Autodesk Fusion 360 part; units mm, degrees
(part 3 of 3)
sketch "Sketch1 (2)" plane through (0, 0, 12.7) normal (0, 0, 1) x (-1, 0, 0)
  arc A0 (-5.2324, 8.6498) -> (-8.6498, 5.2324) centre (0, 0) ccw
  arc A1 (-10.637, 4.5964) -> (-8.6498, 5.2324) centre (-10.0081, 6.054) ccw
  line L0 (-10.637, 4.5964) -> (-21.9128, 9.4616)
  spline S0 degree 5 poles (-21.9128, 9.4616) (-21.9552, 9.4799) (-22.0407, 9.5141) (-22.1712, 9.5583) (-22.3491, 9.6037) (-22.5768, 9.6426) (-22.8081, 9.6692) (-23.0414, 9.6889) (-23.2758, 9.7048) (-23.5109, 9.7174) (-23.7467, 9.7262) (-23.9837, 9.7295) (-24.2219, 9.7262) (-24.4615, 9.7158) (-24.7023, 9.6987) (-24.9439, 9.6758) (-25.1862, 9.648) (-25.4288, 9.6159) (-25.6717, 9.5798) (-25.9149, 9.5397) (-26.1582, 9.4952) (-26.4018, 9.4462) (-26.6456, 9.3926) (-26.8896, 9.3344) (-27.1337, 9.2719) (-27.3777, 9.2051) (-27.6217, 9.1343) (-27.8655, 9.0596) (-28.109, 8.9811) (-28.3523, 8.8987) (-28.5954, 8.8125) (-28.838, 8.7225) (-29.0803, 8.6286) (-29.3222, 8.531) (-29.5637, 8.4296) (-29.8046, 8.3246) (-30.045, 8.216) (-30.2848, 8.1038) (-30.5239, 7.9882) (-30.7623, 7.869) (-31.0001, 7.7465) (-31.2371, 7.6205) (-31.4733, 7.491) (-31.7087, 7.3583) (-31.9432, 7.2221) (-32.1769, 7.0827) (-32.4096, 6.9401) (-32.6414, 6.7942) (-32.8722, 6.6451) (-33.1019, 6.4928) (-33.3306, 6.3374) (-33.5583, 6.1789) (-33.7848, 6.0173) (-34.0102, 5.8526) (-34.2343, 5.6849) (-34.4573, 5.5142) (-34.6791, 5.3405) (-34.8996, 5.1639) (-35.1188, 4.9843) (-35.3367, 4.8018) (-35.5532, 4.6165) (-35.7684, 4.4283) (-35.9823, 4.2373) (-36.1947, 4.0436) (-36.4056, 3.847) (-36.6151, 3.6477) (-36.823, 3.4457) (-37.0294, 3.241) (-37.2343, 3.0337) (-37.4376, 2.8237) (-37.6393, 2.6111) (-37.7995, 2.4389) (-37.9189, 2.3086) (-37.9982, 2.2212) (-38.0377, 2.1774) knots 0 0 0 0 0 0 0.01428571 0.02857143 0.04285714 0.05714286 0.07142857 0.08571429 0.1 0.11428571 0.12857143 0.14285714 0.15714286 0.17142857 0.18571429 0.2 0.21428571 0.22857143 0.24285714 0.25714286 0.27142857 0.28571429 0.3 0.31428571 0.32857143 0.34285714 0.35714286 0.37142857 0.38571429 0.4 0.41428571 0.42857143 0.44285714 0.45714286 0.47142857 0.48571429 0.5 0.51428571 0.52857143 0.54285714 0.55714286 0.57142857 0.58571429 0.6 0.61428571 0.62857143 0.64285714 0.65714286 0.67142857 0.68571429 0.7 0.71428571 0.72857143 0.74285714 0.75714286 0.77142857 0.78571429 0.8 0.81428571 0.82857143 0.84285714 0.85714286 0.87142857 0.88571429 0.9 0.91428571 0.92857143 0.94285714 0.95714286 0.97142857 0.98571429 1 1 1 1 1 1
  arc A2 (-38.0377, 2.1774) -> (-38.0377, -2.1774) centre (0, 0) ccw
  spline S1 degree 5 poles (-38.0377, -2.1774) (-37.9982, -2.2212) (-37.9189, -2.3086) (-37.7995, -2.4389) (-37.6393, -2.6111) (-37.4376, -2.8237) (-37.2343, -3.0337) (-37.0294, -3.241) (-36.823, -3.4457) (-36.6151, -3.6477) (-36.4056, -3.847) (-36.1947, -4.0436) (-35.9823, -4.2373) (-35.7684, -4.4283) (-35.5532, -4.6165) (-35.3367, -4.8018) (-35.1188, -4.9843) (-34.8996, -5.1639) (-34.6791, -5.3405) (-34.4573, -5.5142) (-34.2343, -5.6849) (-34.0102, -5.8526) (-33.7848, -6.0173) (-33.5583, -6.1789) (-33.3306, -6.3374) (-33.1019, -6.4928) (-32.8722, -6.6451) (-32.6414, -6.7942) (-32.4096, -6.9401) (-32.1769, -7.0827) (-31.9432, -7.2221) (-31.7087, -7.3583) (-31.4733, -7.491) (-31.2371, -7.6205) (-31.0001, -7.7465) (-30.7623, -7.869) (-30.5239, -7.9882) (-30.2848, -8.1038) (-30.045, -8.216) (-29.8046, -8.3246) (-29.5637, -8.4296) (-29.3222, -8.531) (-29.0803, -8.6286) (-28.838, -8.7225) (-28.5954, -8.8125) (-28.3523, -8.8987) (-28.109, -8.9811) (-27.8655, -9.0596) (-27.6217, -9.1343) (-27.3777, -9.2051) (-27.1337, -9.2719) (-26.8896, -9.3344) (-26.6456, -9.3926) (-26.4018, -9.4462) (-26.1582, -9.4952) (-25.9149, -9.5397) (-25.6717, -9.5798) (-25.4288, -9.6159) (-25.1862, -9.648) (-24.9439, -9.6758) (-24.7023, -9.6987) (-24.4615, -9.7158) (-24.2219, -9.7262) (-23.9837, -9.7295) (-23.7467, -9.7262) (-23.5109, -9.7174) (-23.2758, -9.7048) (-23.0414, -9.6889) (-22.8081, -9.6692) (-22.5768, -9.6426) (-22.3491, -9.6037) (-22.1712, -9.5583) (-22.0407, -9.5141) (-21.9552, -9.4799) (-21.9128, -9.4616) knots -1 -1 -1 -1 -1 -1 -0.98571429 -0.97142857 -0.95714286 -0.94285714 -0.92857143 -0.91428571 -0.9 -0.88571429 -0.87142857 -0.85714286 -0.84285714 -0.82857143 -0.81428571 -0.8 -0.78571429 -0.77142857 -0.75714286 -0.74285714 -0.72857143 -0.71428571 -0.7 -0.68571429 -0.67142857 -0.65714286 -0.64285714 -0.62857143 -0.61428571 -0.6 -0.58571429 -0.57142857 -0.55714286 -0.54285714 -0.52857143 -0.51428571 -0.5 -0.48571429 -0.47142857 -0.45714286 -0.44285714 -0.42857143 -0.41428571 -0.4 -0.38571429 -0.37142857 -0.35714286 -0.34285714 -0.32857143 -0.31428571 -0.3 -0.28571429 -0.27142857 -0.25714286 -0.24285714 -0.22857143 -0.21428571 -0.2 -0.18571429 -0.17142857 -0.15714286 -0.14285714 -0.12857143 -0.11428571 -0.1 -0.08571429 -0.07142857 -0.05714286 -0.04285714 -0.02857143 -0.01428571 0 0 0 0 0 0
  line L1 (-21.9128, -9.4616) -> (-10.637, -4.5964)
  arc A3 (-8.6498, -5.2324) -> (-10.637, -4.5964) centre (-10.0081, -6.054) ccw
  arc A4 (-8.6498, -5.2324) -> (-5.2324, -8.6498) centre (0, 0) ccw
  arc A5 (-4.5964, -10.637) -> (-5.2324, -8.6498) centre (-6.054, -10.0081) ccw
  line L2 (-4.5964, -10.637) -> (-9.4616, -21.9128)
  spline S2 degree 5 poles (-9.4616, -21.9128) (-9.4799, -21.9552) (-9.5141, -22.0407) (-9.5583, -22.1712) (-9.6037, -22.3491) (-9.6426, -22.5768) (-9.6692, -22.8081) (-9.6889, -23.0414) (-9.7048, -23.2758) (-9.7174, -23.5109) (-9.7262, -23.7467) (-9.7295, -23.9837) (-9.7262, -24.2219) (-9.7158, -24.4615) (-9.6987, -24.7023) (-9.6758, -24.9439) (-9.648, -25.1862) (-9.6159, -25.4288) (-9.5798, -25.6717) (-9.5397, -25.9149) (-9.4952, -26.1582) (-9.4462, -26.4018) (-9.3926, -26.6456) (-9.3344, -26.8896) (-9.2719, -27.1337) (-9.2051, -27.3777) (-9.1343, -27.6217) (-9.0596, -27.8655) (-8.9811, -28.109) (-8.8987, -28.3523) (-8.8125, -28.5954) (-8.7225, -28.838) (-8.6286, -29.0803) (-8.531, -29.3222) (-8.4296, -29.5637) (-8.3246, -29.8046) (-8.216, -30.045) (-8.1038, -30.2848) (-7.9882, -30.5239) (-7.869, -30.7623) (-7.7465, -31.0001) (-7.6205, -31.2371) (-7.491, -31.4733) (-7.3583, -31.7087) (-7.2221, -31.9432) (-7.0827, -32.1769) (-6.9401, -32.4096) (-6.7942, -32.6414) (-6.6451, -32.8722) (-6.4928, -33.1019) (-6.3374, -33.3306) (-6.1789, -33.5583) (-6.0173, -33.7848) (-5.8526, -34.0102) (-5.6849, -34.2343) (-5.5142, -34.4573) (-5.3405, -34.6791) (-5.1639, -34.8996) (-4.9843, -35.1188) (-4.8018, -35.3367) (-4.6165, -35.5532) (-4.4283, -35.7684) (-4.2373, -35.9823) (-4.0436, -36.1947) (-3.847, -36.4056) (-3.6477, -36.6151) (-3.4457, -36.823) (-3.241, -37.0294) (-3.0337, -37.2343) (-2.8237, -37.4376) (-2.6111, -37.6393) (-2.4389, -37.7995) (-2.3086, -37.9189) (-2.2212, -37.9982) (-2.1774, -38.0377) knots 0 0 0 0 0 0 0.01428571 0.02857143 0.04285714 0.05714286 0.07142857 0.08571429 0.1 0.11428571 0.12857143 0.14285714 0.15714286 0.17142857 0.18571429 0.2 0.21428571 0.22857143 0.24285714 0.25714286 0.27142857 0.28571429 0.3 0.31428571 0.32857143 0.34285714 0.35714286 0.37142857 0.38571429 0.4 0.41428571 0.42857143 0.44285714 0.45714286 0.47142857 0.48571429 0.5 0.51428571 0.52857143 0.54285714 0.55714286 0.57142857 0.58571429 0.6 0.61428571 0.62857143 0.64285714 0.65714286 0.67142857 0.68571429 0.7 0.71428571 0.72857143 0.74285714 0.75714286 0.77142857 0.78571429 0.8 0.81428571 0.82857143 0.84285714 0.85714286 0.87142857 0.88571429 0.9 0.91428571 0.92857143 0.94285714 0.95714286 0.97142857 0.98571429 1 1 1 1 1 1
  arc A6 (-2.1774, -38.0377) -> (2.1774, -38.0377) centre (0, 0) ccw
  spline S3 degree 5 poles (2.1774, -38.0377) (2.2212, -37.9982) (2.3086, -37.9189) (2.4389, -37.7995) (2.6111, -37.6393) (2.8237, -37.4376) (3.0337, -37.2343) (3.241, -37.0294) (3.4457, -36.823) (3.6477, -36.6151) (3.847, -36.4056) (4.0436, -36.1947) (4.2373, -35.9823) (4.4283, -35.7684) (4.6165, -35.5532) (4.8018, -35.3367) (4.9843, -35.1188) (5.1639, -34.8996) (5.3405, -34.6791) (5.5142, -34.4573) (5.6849, -34.2343) (5.8526, -34.0102) (6.0173, -33.7848) (6.1789, -33.5583) (6.3374, -33.3306) (6.4928, -33.1019) (6.6451, -32.8722) (6.7942, -32.6414) (6.9401, -32.4096) (7.0827, -32.1769) (7.2221, -31.9432) (7.3583, -31.7087) (7.491, -31.4733) (7.6205, -31.2371) (7.7465, -31.0001) (7.869, -30.7623) (7.9882, -30.5239) (8.1038, -30.2848) (8.216, -30.045) (8.3246, -29.8046) (8.4296, -29.5637) (8.531, -29.3222) (8.6286, -29.0803) (8.7225, -28.838) (8.8125, -28.5954) (8.8987, -28.3523) (8.9811, -28.109) (9.0596, -27.8655) (9.1343, -27.6217) (9.2051, -27.3777) (9.2719, -27.1337) (9.3344, -26.8896) (9.3926, -26.6456) (9.4462, -26.4018) (9.4952, -26.1582) (9.5397, -25.9149) (9.5798, -25.6717) (9.6159, -25.4288) (9.648, -25.1862) (9.6758, -24.9439) (9.6987, -24.7023) (9.7158, -24.4615) (9.7262, -24.2219) (9.7295, -23.9837) (9.7262, -23.7467) (9.7174, -23.5109) (9.7048, -23.2758) (9.6889, -23.0414) (9.6692, -22.8081) (9.6426, -22.5768) (9.6037, -22.3491) (9.5583, -22.1712) (9.5141, -22.0407) (9.4799, -21.9552) (9.4616, -21.9128) knots -1 -1 -1 -1 -1 -1 -0.98571429 -0.97142857 -0.95714286 -0.94285714 -0.92857143 -0.91428571 -0.9 -0.88571429 -0.87142857 -0.85714286 -0.84285714 -0.82857143 -0.81428571 -0.8 -0.78571429 -0.77142857 -0.75714286 -0.74285714 -0.72857143 -0.71428571 -0.7 -0.68571429 -0.67142857 -0.65714286 -0.64285714 -0.62857143 -0.61428571 -0.6 -0.58571429 -0.57142857 -0.55714286 -0.54285714 -0.52857143 -0.51428571 -0.5 -0.48571429 -0.47142857 -0.45714286 -0.44285714 -0.42857143 -0.41428571 -0.4 -0.38571429 -0.37142857 -0.35714286 -0.34285714 -0.32857143 -0.31428571 -0.3 -0.28571429 -0.27142857 -0.25714286 -0.24285714 -0.22857143 -0.21428571 -0.2 -0.18571429 -0.17142857 -0.15714286 -0.14285714 -0.12857143 -0.11428571 -0.1 -0.08571429 -0.07142857 -0.05714286 -0.04285714 -0.02857143 -0.01428571 0 0 0 0 0 0
  line L3 (9.4616, -21.9128) -> (4.5964, -10.637)
  arc A7 (5.2324, -8.6498) -> (4.5964, -10.637) centre (6.054, -10.0081) ccw
  arc A8 (5.2324, -8.6498) -> (8.6498, -5.2324) centre (0, 0) ccw
  arc A9 (10.637, -4.5964) -> (8.6498, -5.2324) centre (10.0081, -6.054) ccw
  line L4 (10.637, -4.5964) -> (21.9128, -9.4616)
  spline S4 degree 5 poles (21.9128, -9.4616) (21.9552, -9.4799) (22.0407, -9.5141) (22.1712, -9.5583) (22.3491, -9.6037) (22.5768, -9.6426) (22.8081, -9.6692) (23.0414, -9.6889) (23.2758, -9.7048) (23.5109, -9.7174) (23.7467, -9.7262) (23.9837, -9.7295) (24.2219, -9.7262) (24.4615, -9.7158) (24.7023, -9.6987) (24.9439, -9.6758) (25.1862, -9.648) (25.4288, -9.6159) (25.6717, -9.5798) (25.9149, -9.5397) (26.1582, -9.4952) (26.4018, -9.4462) (26.6456, -9.3926) (26.8896, -9.3344) (27.1337, -9.2719) (27.3777, -9.2051) (27.6217, -9.1343) (27.8655, -9.0596) (28.109, -8.9811) (28.3523, -8.8987) (28.5954, -8.8125) (28.838, -8.7225) (29.0803, -8.6286) (29.3222, -8.531) (29.5637, -8.4296) (29.8046, -8.3246) (30.045, -8.216) (30.2848, -8.1038) (30.5239, -7.9882) (30.7623, -7.869) (31.0001, -7.7465) (31.2371, -7.6205) (31.4733, -7.491) (31.7087, -7.3583) (31.9432, -7.2221) (32.1769, -7.0827) (32.4096, -6.9401) (32.6414, -6.7942) (32.8722, -6.6451) (33.1019, -6.4928) (33.3306, -6.3374) (33.5583, -6.1789) (33.7848, -6.0173) (34.0102, -5.8526) (34.2343, -5.6849) (34.4573, -5.5142) (34.6791, -5.3405) (34.8996, -5.1639) (35.1188, -4.9843) (35.3367, -4.8018) (35.5532, -4.6165) (35.7684, -4.4283) (35.9823, -4.2373) (36.1947, -4.0436) (36.4056, -3.847) (36.6151, -3.6477) (36.823, -3.4457) (37.0294, -3.241) (37.2343, -3.0337) (37.4376, -2.8237) (37.6393, -2.6111) (37.7995, -2.4389) (37.9189, -2.3086) (37.9982, -2.2212) (38.0377, -2.1774) knots 0 0 0 0 0 0 0.01428571 0.02857143 0.04285714 0.05714286 0.07142857 0.08571429 0.1 0.11428571 0.12857143 0.14285714 0.15714286 0.17142857 0.18571429 0.2 0.21428571 0.22857143 0.24285714 0.25714286 0.27142857 0.28571429 0.3 0.31428571 0.32857143 0.34285714 0.35714286 0.37142857 0.38571429 0.4 0.41428571 0.42857143 0.44285714 0.45714286 0.47142857 0.48571429 0.5 0.51428571 0.52857143 0.54285714 0.55714286 0.57142857 0.58571429 0.6 0.61428571 0.62857143 0.64285714 0.65714286 0.67142857 0.68571429 0.7 0.71428571 0.72857143 0.74285714 0.75714286 0.77142857 0.78571429 0.8 0.81428571 0.82857143 0.84285714 0.85714286 0.87142857 0.88571429 0.9 0.91428571 0.92857143 0.94285714 0.95714286 0.97142857 0.98571429 1 1 1 1 1 1
  arc A10 (38.0377, -2.1774) -> (38.0377, 2.1774) centre (0, 0) ccw
  spline S5 degree 5 poles (38.0377, 2.1774) (37.9982, 2.2212) (37.9189, 2.3086) (37.7995, 2.4389) (37.6393, 2.6111) (37.4376, 2.8237) (37.2343, 3.0337) (37.0294, 3.241) (36.823, 3.4457) (36.6151, 3.6477) (36.4056, 3.847) (36.1947, 4.0436) (35.9823, 4.2373) (35.7684, 4.4283) (35.5532, 4.6165) (35.3367, 4.8018) (35.1188, 4.9843) (34.8996, 5.1639) (34.6791, 5.3405) (34.4573, 5.5142) (34.2343, 5.6849) (34.0102, 5.8526) (33.7848, 6.0173) (33.5583, 6.1789) (33.3306, 6.3374) (33.1019, 6.4928) (32.8722, 6.6451) (32.6414, 6.7942) (32.4096, 6.9401) (32.1769, 7.0827) (31.9432, 7.2221) (31.7087, 7.3583) (31.4733, 7.491) (31.2371, 7.6205) (31.0001, 7.7465) (30.7623, 7.869) (30.5239, 7.9882) (30.2848, 8.1038) (30.045, 8.216) (29.8046, 8.3246) (29.5637, 8.4296) (29.3222, 8.531) (29.0803, 8.6286) (28.838, 8.7225) (28.5954, 8.8125) (28.3523, 8.8987) (28.109, 8.9811) (27.8655, 9.0596) (27.6217, 9.1343) (27.3777, 9.2051) (27.1337, 9.2719) (26.8896, 9.3344) (26.6456, 9.3926) (26.4018, 9.4462) (26.1582, 9.4952) (25.9149, 9.5397) (25.6717, 9.5798) (25.4288, 9.6159) (25.1862, 9.648) (24.9439, 9.6758) (24.7023, 9.6987) (24.4615, 9.7158) (24.2219, 9.7262) (23.9837, 9.7295) (23.7467, 9.7262) (23.5109, 9.7174) (23.2758, 9.7048) (23.0414, 9.6889) (22.8081, 9.6692) (22.5768, 9.6426) (22.3491, 9.6037) (22.1712, 9.5583) (22.0407, 9.5141) (21.9552, 9.4799) (21.9128, 9.4616) knots -1 -1 -1 -1 -1 -1 -0.98571429 -0.97142857 -0.95714286 -0.94285714 -0.92857143 -0.91428571 -0.9 -0.88571429 -0.87142857 -0.85714286 -0.84285714 -0.82857143 -0.81428571 -0.8 -0.78571429 -0.77142857 -0.75714286 -0.74285714 -0.72857143 -0.71428571 -0.7 -0.68571429 -0.67142857 -0.65714286 -0.64285714 -0.62857143 -0.61428571 -0.6 -0.58571429 -0.57142857 -0.55714286 -0.54285714 -0.52857143 -0.51428571 -0.5 -0.48571429 -0.47142857 -0.45714286 -0.44285714 -0.42857143 -0.41428571 -0.4 -0.38571429 -0.37142857 -0.35714286 -0.34285714 -0.32857143 -0.31428571 -0.3 -0.28571429 -0.27142857 -0.25714286 -0.24285714 -0.22857143 -0.21428571 -0.2 -0.18571429 -0.17142857 -0.15714286 -0.14285714 -0.12857143 -0.11428571 -0.1 -0.08571429 -0.07142857 -0.05714286 -0.04285714 -0.02857143 -0.01428571 0 0 0 0 0 0
  line L5 (21.9128, 9.4616) -> (10.637, 4.5964)
  arc A11 (8.6498, 5.2324) -> (10.637, 4.5964) centre (10.0081, 6.054) ccw
  arc A12 (8.6498, 5.2324) -> (5.2324, 8.6498) centre (0, 0) ccw
  arc A13 (4.5964, 10.637) -> (5.2324, 8.6498) centre (6.054, 10.0081) ccw
  line L6 (4.5964, 10.637) -> (9.4616, 21.9128)
  spline S6 degree 5 poles (9.4616, 21.9128) (9.4799, 21.9552) (9.5141, 22.0407) (9.5583, 22.1712) (9.6037, 22.3491) (9.6426, 22.5768) (9.6692, 22.8081) (9.6889, 23.0414) (9.7048, 23.2758) (9.7174, 23.5109) (9.7262, 23.7467) (9.7295, 23.9837) (9.7262, 24.2219) (9.7158, 24.4615) (9.6987, 24.7023) (9.6758, 24.9439) (9.648, 25.1862) (9.6159, 25.4288) (9.5798, 25.6717) (9.5397, 25.9149) (9.4952, 26.1582) (9.4462, 26.4018) (9.3926, 26.6456) (9.3344, 26.8896) (9.2719, 27.1337) (9.2051, 27.3777) (9.1343, 27.6217) (9.0596, 27.8655) (8.9811, 28.109) (8.8987, 28.3523) (8.8125, 28.5954) (8.7225, 28.838) (8.6286, 29.0803) (8.531, 29.3222) (8.4296, 29.5637) (8.3246, 29.8046) (8.216, 30.045) (8.1038, 30.2848) (7.9882, 30.5239) (7.869, 30.7623) (7.7465, 31.0001) (7.6205, 31.2371) (7.491, 31.4733) (7.3583, 31.7087) (7.2221, 31.9432) (7.0827, 32.1769) (6.9401, 32.4096) (6.7942, 32.6414) (6.6451, 32.8722) (6.4928, 33.1019) (6.3374, 33.3306) (6.1789, 33.5583) (6.0173, 33.7848) (5.8526, 34.0102) (5.6849, 34.2343) (5.5142, 34.4573) (5.3405, 34.6791) (5.1639, 34.8996) (4.9843, 35.1188) (4.8018, 35.3367) (4.6165, 35.5532) (4.4283, 35.7684) (4.2373, 35.9823) (4.0436, 36.1947) (3.847, 36.4056) (3.6477, 36.6151) (3.4457, 36.823) (3.241, 37.0294) (3.0337, 37.2343) (2.8237, 37.4376) (2.6111, 37.6393) (2.4389, 37.7995) (2.3086, 37.9189) (2.2212, 37.9982) (2.1774, 38.0377) knots 0 0 0 0 0 0 0.01428571 0.02857143 0.04285714 0.05714286 0.07142857 0.08571429 0.1 0.11428571 0.12857143 0.14285714 0.15714286 0.17142857 0.18571429 0.2 0.21428571 0.22857143 0.24285714 0.25714286 0.27142857 0.28571429 0.3 0.31428571 0.32857143 0.34285714 0.35714286 0.37142857 0.38571429 0.4 0.41428571 0.42857143 0.44285714 0.45714286 0.47142857 0.48571429 0.5 0.51428571 0.52857143 0.54285714 0.55714286 0.57142857 0.58571429 0.6 0.61428571 0.62857143 0.64285714 0.65714286 0.67142857 0.68571429 0.7 0.71428571 0.72857143 0.74285714 0.75714286 0.77142857 0.78571429 0.8 0.81428571 0.82857143 0.84285714 0.85714286 0.87142857 0.88571429 0.9 0.91428571 0.92857143 0.94285714 0.95714286 0.97142857 0.98571429 1 1 1 1 1 1
  arc A14 (2.1774, 38.0377) -> (-2.1774, 38.0377) centre (0, 0) ccw
  spline S7 degree 5 poles (-2.1774, 38.0377) (-2.2212, 37.9982) (-2.3086, 37.9189) (-2.4389, 37.7995) (-2.6111, 37.6393) (-2.8237, 37.4376) (-3.0337, 37.2343) (-3.241, 37.0294) (-3.4457, 36.823) (-3.6477, 36.6151) (-3.847, 36.4056) (-4.0436, 36.1947) (-4.2373, 35.9823) (-4.4283, 35.7684) (-4.6165, 35.5532) (-4.8018, 35.3367) (-4.9843, 35.1188) (-5.1639, 34.8996) (-5.3405, 34.6791) (-5.5142, 34.4573) (-5.6849, 34.2343) (-5.8526, 34.0102) (-6.0173, 33.7848) (-6.1789, 33.5583) (-6.3374, 33.3306) (-6.4928, 33.1019) (-6.6451, 32.8722) (-6.7942, 32.6414) (-6.9401, 32.4096) (-7.0827, 32.1769) (-7.2221, 31.9432) (-7.3583, 31.7087) (-7.491, 31.4733) (-7.6205, 31.2371) (-7.7465, 31.0001) (-7.869, 30.7623) (-7.9882, 30.5239) (-8.1038, 30.2848) (-8.216, 30.045) (-8.3246, 29.8046) (-8.4296, 29.5637) (-8.531, 29.3222) (-8.6286, 29.0803) (-8.7225, 28.838) (-8.8125, 28.5954) (-8.8987, 28.3523) (-8.9811, 28.109) (-9.0596, 27.8655) (-9.1343, 27.6217) (-9.2051, 27.3777) (-9.2719, 27.1337) (-9.3344, 26.8896) (-9.3926, 26.6456) (-9.4462, 26.4018) (-9.4952, 26.1582) (-9.5397, 25.9149) (-9.5798, 25.6717) (-9.6159, 25.4288) (-9.648, 25.1862) (-9.6758, 24.9439) (-9.6987, 24.7023) (-9.7158, 24.4615) (-9.7262, 24.2219) (-9.7295, 23.9837) (-9.7262, 23.7467) (-9.7174, 23.5109) (-9.7048, 23.2758) (-9.6889, 23.0414) (-9.6692, 22.8081) (-9.6426, 22.5768) (-9.6037, 22.3491) (-9.5583, 22.1712) (-9.5141, 22.0407) (-9.4799, 21.9552) (-9.4616, 21.9128) knots -1 -1 -1 -1 -1 -1 -0.98571429 -0.97142857 -0.95714286 -0.94285714 -0.92857143 -0.91428571 -0.9 -0.88571429 -0.87142857 -0.85714286 -0.84285714 -0.82857143 -0.81428571 -0.8 -0.78571429 -0.77142857 -0.75714286 -0.74285714 -0.72857143 -0.71428571 -0.7 -0.68571429 -0.67142857 -0.65714286 -0.64285714 -0.62857143 -0.61428571 -0.6 -0.58571429 -0.57142857 -0.55714286 -0.54285714 -0.52857143 -0.51428571 -0.5 -0.48571429 -0.47142857 -0.45714286 -0.44285714 -0.42857143 -0.41428571 -0.4 -0.38571429 -0.37142857 -0.35714286 -0.34285714 -0.32857143 -0.31428571 -0.3 -0.28571429 -0.27142857 -0.25714286 -0.24285714 -0.22857143 -0.21428571 -0.2 -0.18571429 -0.17142857 -0.15714286 -0.14285714 -0.12857143 -0.11428571 -0.1 -0.08571429 -0.07142857 -0.05714286 -0.04285714 -0.02857143 -0.01428571 0 0 0 0 0 0
  line L7 (-9.4616, 21.9128) -> (-4.5964, 10.637)
  arc A15 (-5.2324, 8.6498) -> (-4.5964, 10.637) centre (-6.054, 10.0081) ccw
  circle A16 centre (0, 0) radius 6.35
  circle A17 centre (0, 0) radius 7
  circle A18 centre (0, 0) radius 6.35
  line L8 (1.4, -6.8586) -> (1.4, -5.1)
  line L9 (1.4, -5.1) -> (-1.4, -5.1)
  line L10 (-1.4, -5.1) -> (-1.4, -6.8586)
  line L11 (0, -9) -> (0, 8.2774)
  point P0 (0, -7)
  dimension "d17" = 14
  dimension "d18" = 2.8
  dimension "d19" = 1.9
  constraint coincident A0.centre A2.centre
  constraint coincident A17 L8.start
  constraint vertical L8
  constraint perpendicular L8 L9
  constraint coincident A17 L10.end
  constraint perpendicular L9 L10
  constraint perpendicular L9 L11
  constraint symmetric L8 L10 L11
  constraint coincident A17 P0
  constraint coincident L11 P0
  constraint coincident A0.centre L11
  measures "d17" diameter of A17
  measures "d18" distance of L8 L10
  measures "d19" distance of L9 P0
extrude "Extrude3" cut sketch "Sketch1 (2)" against normal blind 12.7 contours A16 A17 A18 L8 L11 | A16 A17 A18 L10 L11 | A16 A17 A18 L8 L11 | A16 A17 A18 L10 L11 in component "Spur Gear (4 teeth)"
extrude "Extrude4" add sketch "Sketch1 (2)" against normal up to surface (12.7 mm away) contours A16 A17 A18 L8 L11 | A16 A18 L8 L9 L11 | A16 A18 L9 L10 L11 | A16 A17 A18 L10 L11 picked at (1.2459, -6.4442) picked at (0.7792, -5.4935) picked at (-0.7792, -5.4935) picked at (-1.2459, -6.4442) in component "Spur Gear (4 teeth)"
component "Spur Gear (4 teeth)" placed x (1, 0, 0) y (0, 1, 0) z (0, 0, 1) at (0, 0, 0)

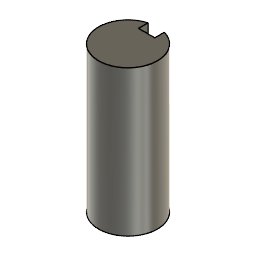
design "Motor Shaft"
Autodesk Fusion 360 part; units mm, degrees
sketch "Sketch1" plane through (0, 0, 0) normal (0, 0, 1) x (1, 0, 0)
  circle A0 centre (0, 0) radius 5.45
  line L0 (0, 7.5) -> (0, -6)
  line L1 (-1.5, 5.2395) -> (-1.5, 3.45)
  line L2 (-1.5, 3.45) -> (1.5, 3.45)
  line L3 (1.5, 3.45) -> (1.5, 5.2395)
  circle A1 centre (0, 0) radius 3.2
  line L4 (-2.0805, -2.4314) -> (2.0805, -2.4314)
  point P0 (0, 5.45)
  dimension "d1" = 10.9
  dimension "d2" = 2
  dimension "d3" = 3
  dimension "d4" = 6.4
  dimension "d5" = 4.161
  constraint coincident A0.centre A1.centre
  constraint vertical L0
  constraint coincident A0 L1.start
  constraint parallel L0 L1
  constraint perpendicular L1 L2
  constraint coincident A0 L3.end
  constraint perpendicular L2 L3
  constraint symmetric L0 L1 L3
  constraint coincident A0 P0
  constraint coincident L0 P0
  constraint coincident A0.centre L0
  constraint coincident A1 L4.start
  constraint coincident A1 L4.end
  constraint perpendicular L0 L4
  measures "d1" diameter of A0
  measures "d2" distance of L2 P0
  measures "d3" distance of L1 L3
  measures "d4" diameter of A1
  measures "d5" distance of L4.start L4.end
extrude "Extrude1" add sketch "Sketch1" along normal blind 15
extrude "Extrude2" add sketch "Sketch1" against normal blind 12 contours A0 L0 L2 L3 A1 | A0 L0 L2 L3 | A0 L0 L1 L2 A1 | A0 L0 L1 L2 | L0 A1 L4 | L0 A1 L4 picked at (-0.1505, -2.9331) picked at (0.1505, -2.9331)
extrude "Extrude3" cut sketch "Sketch1" against normal blind 10 from surface at 15 contours A0 L0 L2 L3 | A0 L0 L1 L2

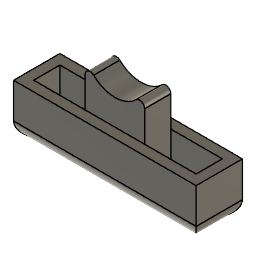
design "Cap 3"
Autodesk Fusion 360 part; units mm, degrees
sketch "Sketch1" plane through (0, 0, 0) normal (0, 0, 1) x (1, 0, 0)
  line L0 (0, 0) -> (32.2, 0)
  line L1 (32.2, 0) -> (32.2, 5.2)
  line L2 (32.2, 5.2) -> (0, 5.2)
  line L3 (0, 5.2) -> (0, 0)
  line L4 (-2, -2) -> (34.2, -2)
  line L5 (34.2, -2) -> (34.2, 7.2)
  line L6 (34.2, 7.2) -> (-2, 7.2)
  line L7 (-2, 7.2) -> (-2, -2)
  line L8 (10.2, 5.2) -> (22, 5.2)
  line L9 (22, 5.2) -> (22, 0)
  line L10 (22, 0) -> (10.2, 0)
  line L11 (10.2, 0) -> (10.2, 5.2)
  dimension "d1" = 5.2
  dimension "d2" = 32.2
  dimension "d3" = 2
  dimension "d4" = 10.2
  dimension "d5" = 10.2
  constraint horizontal L0
  constraint vertical L1
  constraint horizontal L2
  constraint vertical L3
  constraint coincident L0.start L3.end
  constraint horizontal L8
  constraint vertical L9
  constraint horizontal L10
  constraint vertical L11
  constraint coincident L0 L9.end
  constraint coincident L2 L8.start
  measures "d1" distance of L0 L2
  measures "d2" distance of L1 L3
  measures "d4" distance of L3 L11
  measures "d5" distance of L1 L9
extrude "Extrude1" add sketch "Sketch1" along normal blind 8
extrude "Extrude2" add sketch "Sketch1" against normal blind 2 contours L0 L2 L3 L11 | L0 L2 L8 L9 L10 L11 | L0 L1 L2 L9 | L4 L5 L6 L7
extrude "Extrude3" add sketch "Sketch1" along normal blind 18 contours L0 L2 L8 L9 L10 L11
sketch "Sketch2" plane through (0, 5.2, 0) normal (0, 1, 0) x (-1, 0, 0)
  line L0 (-22, 8) -> (-10.2, 8)
  line L1 (-10.2, 8) -> (-10.2, 18)
  line L2 (-10.2, 18) -> (-22, 18)
  line L3 (-22, 18) -> (-22, 8)
  arc A0 (-22, 18) -> (-10.2, 18) centre (-16.1, 19.0909) ccw
  dimension "d19" = 6
  constraint coincident L2.end L3.start
  constraint coincident L1.end L2.start
  measures "d19" radius of A0
extrude "Extrude4" cut sketch "Sketch2" against normal up to surface (5.2 mm away) contours L2 A0
fillet "Fillet1" radius 3 4 edges at (-2, 2.6, -2) (16.1, 7.2, -2) (34.2, 2.6, -2) (16.1, -2, -2)
fillet "Fillet3" radius 1 2 edges at (10.2, 2.6, 18) (22, 2.6, 18)

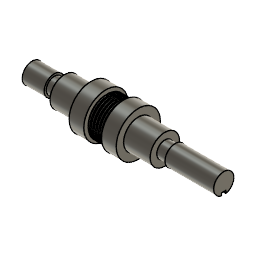
design "Roller 1"
Autodesk Fusion 360 part; units mm, degrees
sketch "Sketch1" plane through (0, 0, 0) normal (1, 0, 0) x (0, 1, 0)
  circle A0 centre (0, 0) radius 10
  circle A1 centre (0, 0) radius 5.5
  circle A2 centre (0, 0) radius 6.9
  line L0 (-1.5, -6.735) -> (-1.5, -4.9)
  line L1 (-1.5, -4.9) -> (1.5, -4.9)
  line L2 (1.5, -4.9) -> (1.5, -6.735)
  line L3 (0, -11) -> (0, 11)
  line L4 (1.0311, 3.6) -> (1.4, 3.6)
  line L5 (1.4, 3.6) -> (1.4, 5.3188)
  line L6 (-1.0311, 3.6) -> (-1.4, 3.6)
  line L7 (-1.4, 3.6) -> (-1.4, 5.3188)
  line L8 (1.0311, 3.6) -> (-1.0311, 3.6)
  circle A3 centre (0, 0) radius 7.9
  circle A4 centre (0, 0) radius 15
  circle A5 centre (0, 0) radius 13
  circle A6 centre (0, 0) radius 12
  point P0 (0, -6.9)
  point P1 (0, 5.5)
  dimension "d1" = 20
  dimension "d4" = -4.5
  dimension "d11" = 13.8
  dimension "d15" = 3
  dimension "d16" = 2
  dimension "d31" = 2.8
  dimension "d32" = 1.9
  dimension "d55" = 1
  dimension "d56" = 5
  dimension "d57" = -2
  dimension "d58" = -1
  constraint coincident A0.centre A1.centre
  constraint coincident A2 L0.start
  constraint vertical L0
  constraint perpendicular L0 L1
  constraint coincident A2 L2.end
  constraint perpendicular L1 L2
  constraint vertical L3
  constraint symmetric L0 L2 L3
  constraint coincident A2 P0
  constraint coincident L3 P0
  constraint coincident A0.centre L3
  constraint horizontal L4
  constraint vertical L5
  constraint coincident A1 L5.end
  constraint horizontal L6
  constraint vertical L7
  constraint coincident A1 L7.end
  constraint perpendicular L3 L8
  constraint coincident L3 P1
  constraint coincident A1 P1
  constraint symmetric L3 L5 L7
  measures "d1" diameter of A0
  measures "d11" diameter of A2
  measures "d15" distance of L0 L2
  measures "d16" distance of L1 P0
  measures "d31" distance of L5 L7
  measures "d32" distance of L8 P1
extrude "Extrude1" add sketch "Sketch1" along normal blind 130 contours A0 L3 A3 | A0 L3 A3 | A2 L3 A3 | A2 L3 A3 | A1 A2 L0 L3 | A1 A2 L2 L3 | A1 A2 L2 L3 | A1 A2 L0 L3 | A1 L3 L6 L7 L8 | A1 L3 L4 L5 L8 | A1 L1 L2 L3 | A1 L0 L1 L3 | A1 L0 L1 L3 L6 L7 L8 | A1 L1 L2 L3 L4 L5 L8
extrude "Extrude2" cut sketch "Sketch1" along normal blind 7 from surface at 15 contours A0 L3 A3 | A0 L3 A3 | A2 L3 A3 | A2 L3 A3 | A1 A2 L0 L3 | A1 A2 L2 L3 | A1 A2 L2 L3 | A1 A2 L0 L3
extrude "Extrude3" cut sketch "Sketch1" along normal blind 7 from surface at 90 contours A0 L3 A3 | A0 L3 A3 | A2 L3 A3 | A2 L3 A3 | A1 A2 L0 L3 | A1 A2 L2 L3 | A1 A2 L2 L3 | A1 A2 L0 L3
extrude "Extrude4" cut sketch "Sketch1" along normal up to surface (33 mm away) from surface at 97 contours A0 L3 A3 | A0 L3 A3 | A2 L3 A3 | A2 L3 A3
extrude "Extrude5" cut sketch "Sketch1" along normal up to surface (24 mm away) from surface at 106 contours A1 A2 L2 L3 | A1 A2 L0 L3 | A1 L1 L2 L3 | A1 L0 L1 L3 picked at (0.8391, -5.9034) picked at (-0.8391, -5.9034)
extrude "Extrude6" cut sketch "Sketch1" along normal up to surface (15 mm away) contours A0 L3 A3 | A0 L3 A3 | A2 L3 A3 | A2 L3 A3
extrude "Extrude7" add sketch "Sketch1" along normal blind 32 from surface at 40 contours A4 | A5 | A6
extrude "Extrude8" cut sketch "Sketch1" along normal blind 10 contours A1 L1 L2 L3 | A1 L0 L1 L3 | A1 L0 L1 L3 L6 L7 L8 | A1 L1 L2 L3 L4 L5 L8
extrude "Extrude9" cut sketch "Sketch1" along normal blind 12 from surface at 50 contours A4
extrude "Extrude15" cut sketch "Sketch1" along normal blind 1 from surface at 50 contours A5
extrude "Extrude16" cut sketch "Sketch1" along normal blind 1 from surface at 52 contours A5
extrude "Extrude17" cut sketch "Sketch1" along normal blind 1 from surface at 54 contours A5
extrude "Extrude18" cut sketch "Sketch1" along normal blind 1 from surface at 56 contours A5
extrude "Extrude19" cut sketch "Sketch1" along normal blind 1 from surface at 58 contours A5
extrude "Extrude20" cut sketch "Sketch1" along normal blind 1 from surface at 60 contours A5

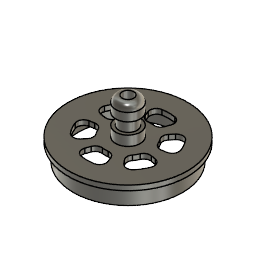
design "Back Reel Shaft"
Autodesk Fusion 360 part; units mm, degrees
sketch "Sketch1" plane through (0, 0, 0) normal (0, 0, 1) x (1, 0, 0)
  circle A0 centre (0, 0) radius 30.4
  circle A1 centre (0, 0) radius 33.4
  circle A2 centre (0, 0) radius 36.4
  circle A3 centre (0, 0) radius 7.5
  circle A4 centre (0, 0) radius 14
  line L0 (0, 0) -> (4.7883, -13.1557)
  line L1 (0, 0) -> (-4.7883, -13.1557)
  line L2 (0, -60) -> (0, 60)
  line L3 (4.7883, -13.1557) -> (8.5505, -23.4923)
  line L4 (-4.7883, -13.1557) -> (-8.5505, -23.4923)
  arc A5 (8.5505, -23.4923) -> (-8.5505, -23.4923) centre (0, 0) ccw
  arc A6 (-8.5505, -23.4923) -> (0, -25) centre (0, 0) ccw
  arc A7 (0, -25) -> (8.5505, -23.4923) centre (0, 0) ccw
  line L5 (13.7873, -2.4311) -> (24.6202, -4.3412)
  line L6 (8.999, -10.7246) -> (16.0697, -19.1511)
  line L7 (8.999, 10.7246) -> (16.0697, 19.1511)
  line L8 (13.7873, 2.4311) -> (24.6202, 4.3412)
  line L9 (-4.7883, 13.1557) -> (-8.5505, 23.4923)
  line L10 (4.7883, 13.1557) -> (8.5505, 23.4923)
  line L11 (-13.7873, 2.4311) -> (-24.6202, 4.3412)
  line L12 (-8.999, 10.7246) -> (-16.0697, 19.1511)
  line L13 (-8.999, -10.7246) -> (-16.0697, -19.1511)
  line L14 (-13.7873, -2.4311) -> (-24.6202, -4.3412)
  circle A8 centre (0, 0) radius 3.5
  circle A9 centre (0, 0) radius 5.5
  point P0 (0, 7.5)
  dimension "d1" = 60.8
  dimension "d2" = 3
  dimension "d3" = 3
  dimension "d4" = 15
  dimension "d11" = 28
  dimension "d12" = 50
  dimension "d13" = 40
  dimension "d15" = 20
  dimension "d17" = 360
  dimension "d22" = -4
  dimension "d34" = -2
  constraint coincident A0.centre A1.centre
  constraint concentric A0 A3
  constraint concentric A0 A5
  constraint concentric A0 A4
  constraint vertical L2
  constraint coincident A4 L0.end
  constraint coincident A4 L1.end
  constraint coincident L2 A6.end
  constraint concentric A5 A6
  constraint concentric A5 A7
  constraint coincident A3 P0
  constraint coincident L2 P0
  constraint coincident A0.centre L2
  measures "d1" diameter of A0
  measures "d4" diameter of A3
  measures "d11" diameter of A4
  measures "d12" diameter of A5
  measures "d13" angle of L0 L1
  measures "d15" angle of L1 L2
extrude "Extrude1" add sketch "Sketch1" against normal blind 10 contours A0 A1 L2 | A0 A1 L2
extrude "Extrude2" add sketch "Sketch1" along normal blind 3
extrude "Extrude3" add sketch "Sketch1" along normal blind 25 contours A3 L1 L2 A9 | A3 L0 L2 A9 | A3 L0 L2 A9 | A3 L1 L2 A9 | L0 L2 A8 A9 | L1 L2 A8 A9 | L1 L2 A8 A9 | L0 L2 A8 A9 | L0 L2 A8 | L1 L2 A8 | L1 L2 A8 | L0 L2 A8
extrude "Extrude4" cut sketch "Sketch1" along normal blind 3 contours A4 L2 A5 L10 | A4 L2 A5 L9 | A4 L2 L4 A6 | A4 L2 L3 A7 | A4 A5 L7 L8 | A4 A5 L11 L12 | A4 A5 L13 L14 | A4 A5 L5 L6
fillet "Fillet1" radius 4 24 edges at (-16.0697, 19.1511, 1.5) (-24.6202, 4.3412, 1.5) (-13.7873, 2.4311, 1.5) (-8.999, 10.7246, 1.5) (-13.7873, -2.4311, 1.5) (-24.6202, -4.3412, 1.5) (-16.0697, -19.1511, 1.5) (-8.999, -10.7246, 1.5) (-4.7883, -13.1557, 1.5) (-8.5505, -23.4923, 1.5) (8.5505, -23.4923, 1.5) (4.7883, -13.1557, 1.5) (8.999, -10.7246, 1.5) (16.0697, -19.1511, 1.5) (24.6202, -4.3412, 1.5) (13.7873, -2.4311, 1.5) (24.6202, 4.3412, 1.5) (16.0697, 19.1511, 1.5) (13.7873, 2.4311, 1.5) (8.999, 10.7246, 1.5) (4.7883, 13.1557, 1.5) (8.5505, 23.4923, 1.5) (-4.7883, 13.1557, 1.5) (-8.5505, 23.4923, 1.5)
extrude "Extrude5" cut sketch "Sketch1" against normal up to surface (22 mm away) from surface at 25 contours L0 L2 A8 | L1 L2 A8 | L1 L2 A8 | L0 L2 A8
extrude "Extrude7" cut sketch "Sketch1" along normal blind 7 from surface at 9 contours A3 L1 L2 A9 | A3 L0 L2 A9 | A3 L0 L2 A9 | A3 L1 L2 A9
fillet "Fillet4" radius 4 1 edges at (-6.9925, -2.7121, 25)

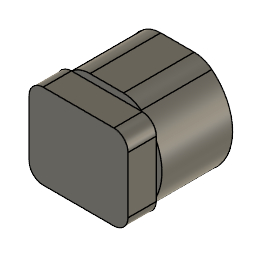
design "Sleeve"
Autodesk Fusion 360 part; units mm, degrees
sketch "Sketch1" plane through (0, 0, 0) normal (0, 0, 1) x (1, 0, 0)
  line L0 (0, 0) -> (7, 0)
  line L1 (7, 0) -> (7, 2)
  line L2 (7, 2) -> (0, 2)
  line L3 (0, 2) -> (0, 0)
  dimension "d1" = 7
  dimension "d2" = 2
  constraint horizontal L0
  constraint vertical L1
  constraint horizontal L2
  constraint vertical L3
  constraint coincident L0.start L3.end
  measures "d1" distance of L0.start L0.end
  measures "d2" distance of L0 L2
extrude "Extrude1" add sketch "Sketch1" along normal blind 6
sketch "Sketch2" plane through (0, 2, 0) normal (0, 1, 0) x (-1, 0, 0)
  line L0 (-7, 0) -> (0, 0)
  line L1 (0, 0) -> (0, 6)
  line L2 (0, 6) -> (-7, 6)
  line L3 (-7, 6) -> (-7, 0)
  line L4 (-7, 3) -> (0, 3) construction
  line L5 (-3.5, 6) -> (-3.5, 0) construction
  circle A0 centre (-3.5, 3) radius 2.9
  circle A1 centre (-3.5, 3) radius 3.9
  line L6 (-5.2491, -0.4858) -> (-1.7509, -0.4858)
  line L7 (-5.2491, 6.4858) -> (-1.7509, 6.4858)
  dimension "d5" = 5.8
  dimension "d6" = 1
  constraint midpoint L3 L4.start
  constraint midpoint L1 L4.end
  constraint midpoint L2 L5.start
  constraint midpoint L0 L5.end
  constraint midpoint L5 A0.centre
  constraint coincident A1 L6.start
  constraint coincident A1 L6.end
  constraint horizontal L6
  constraint symmetric L4 L6.start L7.start
  constraint symmetric L4 L6.end L7.end
  measures "d5" diameter of A0
extrude "Extrude2" add sketch "Sketch2" along normal blind 5 contours L0 L1 L2 L3 A1 | L0 A1 L6 | L3 A1 | L1 A1 | L2 A1 L7
fillet "Fillet1" radius 1 4 edges at (0, 1, 6) (0, 1, 0) (7, 1, 0) (7, 1, 6)
fillet "Fillet2" radius 2 4 edges at (1.7509, 4.5, 6.4858) (5.2491, 4.5, 6.4858) (5.2491, 4.5, -0.4858) (1.7509, 4.5, -0.4858)
